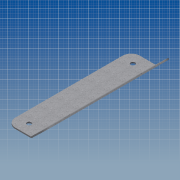
# Autodesk Inventor part: J009600
Saved by Autodesk Inventor 2020.3 (Build 243373000, 373)
## iProperties
RuleStatus: InUse
AfterDocSave0: file://Part Number Cleaner
Created: 2020-12-04
Material: STAINLESS STEEL, 316
Catalog Web Link: https://www.janelia.org/
Vendor: HHMI: JRC - ID&F
Document SubType Name: Sheet Metal
Designer: talbotj
Density: 8 g/cm^3
Sheet Metal Rule: Default
Appearance: Metal-Steel (Stainless, Brushed)
Flat Pattern Width: 3.5469 cm
Flat Pattern Length: 9.144 cm
Flat Pattern Area: 32.4328 cm^2
Sheet Metal Width: 1.396 in
Sheet Metal Length: 3.600 in
Sheet Metal Area: 5.027 in^2
Part Number: J009600
Description: N/A
Project: N/A
DESIGN DEPARTMENT: HHMI: JRC - ID&F
SPECIAL FINISH: N/A
LAB/DEPT: VIVARIUM (SHARED RESOURCES)
REQUESTING SCIENTIST: COX, JAMES
SURFACE ROUGHNESS: N/A
Thickness: 0.036 in
ALTERED ITEM PART NUMBER: N/A
ALTERED ITEM VENDOR: N/A
ALTERED ITEM DESCRIPTION: N/A
PART NUMBER - LEGACY: N/A
Author: talbotj
Revision Number: -
Autodesk Inventor part; units mm, degrees
ref_plane "YZ Plane" through (0, 0, 0) normal (1, 0, 0) x (0, 1, 0)
ref_plane "XZ Plane" through (0, 0, 0) normal (0, 1, 0) x (-1, 0, 0)
ref_plane "XY Plane" through (0, 0, 0) normal (0, 0, 1) x (1, 0, 0)
sketch "Sketch1" plane through (0, 0, 0) normal (0, 1, 0) x (-1, 0, 0)
  line L0 (-8.89, -45.72) -> (8.89, -45.72)
  line L1 (8.89, -45.72) -> (8.89, 45.72)
  line L2 (8.89, 45.72) -> (-8.89, 45.72)
  line L3 (-8.89, 45.72) -> (-8.89, -45.72)
  line L4 (-8.89, -45.72) -> (8.89, 45.72) construction
  line L5 (8.89, -45.72) -> (-8.89, 45.72) construction
  point P0 (0, 0)
  dimension "d0" = 17.78
  dimension "d1" = 91.44
  measures "d0" distance of L2.end L1.end
  measures "d1" distance of L1.end L0.end
extrude "Plate1" add sketch "Sketch1" along normal blind 0.9144
sketch "Sketch2" plane through (8.89, 0.9144, -45.72) normal (0.6946584, -0.7193398, 0) x (0.7193398, 0.6946584, 0)
  line L0 (0, 91.44) -> (0, 0)
  line L1 (0, 0) -> (17.4106, 0)
  line L2 (17.4106, 0) -> (17.4106, 91.44)
  line L3 (17.4106, 91.44) -> (0, 91.44)
  constraints: 6 end point, 1 horizontal, 1 perpendicular, 1 vertical
edge flange "Flange1" height 17.78 angle 44 thickness 0.9144 bend radius 0.762 thickness toward (0.6946584, -0.7193398, 0) relief tear relief width 0.9144 relief depth 0.4572 edges at (8.89, 0.9144, 0) wall of the first edge with corners at (8.89, 0.9144, 45.72) (8.89, 0.9144, -45.72) (21.4141, 13.0088, -45.72) (21.4141, 13.0088, 45.72)
bend "Bend1"
corner "Corner1"
sketch "Sketch3" plane through (0, 0.9144, 0) normal (0, 1, 0) x (1, 0, 0)
  line L0 (-14.9938, 0) -> (27.733, 0) projected
  line L1 (-8.89, -45.72) -> (-8.89, 45.72) projected
  point P0 (0, 0)
  point P1 (0, 38.1)
  point P2 (0, -38.1)
  dimension "d13" = 76.2
  dimension "d14" = 8.89
  constraints: 1 symmetric about line, 1 vertical alignment
  measures "d13" distance of point (0, -38.1) point (0, 38.1)
  measures "d14" distance from line of L1 point (0, 38.1)
hole "Hole1" at (0, 0.9144, -38.1) at (0, 0.9144, 38.1) direction (0, -1, 0) diameter 3.2512 end through all
sketch "Sketch4" plane through (21.4141, 13.0088, -45.72) normal (-0.6946584, 0.7193398, 0) x (0, 0, 1)
  line L0 (91.44, 0) -> (0, 0) projected
  line L1 (45.72, -40.2779) -> (45.72, 7.2461) projected
  point P0 (45.72, -24.4407)
  point P1 (19.304, -7.239)
  point P2 (72.136, -7.239)
  dimension "d22" = 7.239
  dimension "d23" = 52.832
  constraints: 1 horizontal alignment, 1 symmetric about line
  measures "d22" distance from line of L0 point (19.304, -7.239)
  measures "d23" distance of point (72.136, -7.239) point (19.304, -7.239)
hole "Hole2" at (16.2068, 7.9802, -26.416) at (16.2068, 7.9802, 26.416) direction (0.6946584, -0.7193398, 0) diameter 3.2512 end through all
fillet "Corner Round1" radius 6.35 4 edges at (-8.89, 0.4572, 45.72) (21.7317, 12.6799, -45.72) (-8.89, 0.4572, -45.72) (21.7317, 12.6799, 45.72)
equation "\"d20\" = Thickness"
equation "\"d29\" = Thickness"
equation "\"d2\" = Thickness"
equation "\"d3\" = BendReliefWidth"
equation "\"d4\" = BendReliefDepth"
equation "\"d5\" = MinimumRemnant"
equation "\"d6\" = TransitionRadius"
equation "\"d9\" = BendRadius"
equation "\"d10\" = CornerReliefSize"
equation "\"d11\" = GapSize"
equation "\"d12\" = JacobiRadiusSize"
equation "\"BendReliefWidth\" = Thickness"
equation "\"BendReliefDepth\" = 0.5 * Thickness"
equation "\"CornerReliefSize\" = 4 * Thickness"
equation "\"MinimumRemnant\" = 2 * Thickness"
equation "\"TransitionRadius\" = BendRadius"
equation "\"JacobiRadiusSize\" = BendRadius"
equation "\"GapSize\" = Thickness"
equation "\"Thickness\" = 0.9144"
equation "\"BendRadius\" = 0.762"
body "Solid1"
